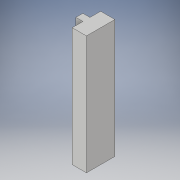
# Autodesk Inventor part: 000.403 - Т-образный стержень
Saved by Autodesk Inventor 2019 (Build 230136000, 136)
## iProperties
Created: 2020-03-21
Part Number: 000.403 - Т-образный стержень
Material: Типовые
Document SubType Name: Modeling
Designer: Петров Иван
Density: 1 g/cm^3
Appearance: По умолчанию
Author: Петров Иван
Autodesk Inventor part; units mm, degrees
ref_plane "YZ Plane" through (0, 0, 0) normal (1, 0, 0) x (0, 1, 0)
ref_plane "XZ Plane" through (0, 0, 0) normal (0, 1, 0) x (-1, 0, 0)
ref_plane "XY Plane" through (0, 0, 0) normal (0, 0, 1) x (1, 0, 0)
sketch "Эскиз1" plane through (0, 0, 0) normal (0, 1, 0) x (-1, 0, 0)
  line L0 (6, 12) -> (-6, 12)
  line L1 (-6, 12) -> (-6, -12)
  line L2 (-6, -12) -> (6, -12)
  line L3 (12, -3) -> (12, 3)
  line L4 (12, 3) -> (6, 3)
  line L5 (6, -3) -> (12, -3)
  line L6 (6, -12) -> (6, -3)
  line L7 (6, 3) -> (6, 12)
  point P0 (0, 0)
  point P1 (0, 0)
  point P2 (0, 0)
  constraints: 16 end point, 4 parallel, 3 perpendicular
extrude "Выдавливание1" add sketch "Эскиз1" along normal blind 100
